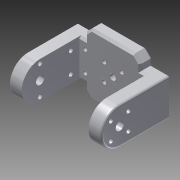
# Autodesk Inventor part: サーボ首不利
Saved by Autodesk Inventor 2015 (Build 190159000, 159)
## iProperties
Created: 2015-05-13
Part Number: サーボ首不利
Material: PVC、軟質
Document SubType Name: Modeling
Designer: kenta
Density: 1.3 g/cm^3
Appearance: PVC - 白
Mass: 15.4827 g
Surface Area: 60.3665 cm^2
Volume: 11.9097 cm^3
Author: kenta
Autodesk Inventor part; units mm, degrees
note: some values were not read from the file. Chosen so that the rebuilt part matches the saved one: direction of "穴4"; direction of "穴5"; direction of "穴6"; direction of "穴7"; direction of "穴8".
ref_plane "YZ Plane" through (0, 0, 0) normal (1, 0, 0) x (0, 1, 0)
ref_plane "XZ Plane" through (0, 0, 0) normal (0, 1, 0) x (-1, 0, 0)
ref_plane "XY Plane" through (0, 0, 0) normal (0, 0, 1) x (1, 0, 0)
sketch "スケッチ1" plane through (0, 0, 0) normal (0, 0, 1) x (1, 0, 0)
  line L0 (-22.5, 17) -> (22.5, 17)
  line L1 (22.5, 17) -> (22.5, -17)
  line L2 (22.5, -17) -> (-22.5, -17)
  line L3 (-22.5, -17) -> (-22.5, 17)
  line L4 (-22.5, 17) -> (22.5, -17) construction
  line L5 (22.5, 17) -> (-22.5, -17) construction
  point P0 (0, 0)
  dimension "d0" = 45
  dimension "d1" = 34
  constraints: 12 end point, 2 midpoint, 2 parallel, 1 horizontal, 1 perpendicular
  measures "d0" distance of L1.end L2.end
  measures "d1" distance of L0.end L1.end
extrude "押し出し1" add sketch "スケッチ1" along normal blind 18
sketch "スケッチ2" plane through (0, 0, 18) normal (0, 0, 1) x (1, 0, 0)
  line L0 (-16.25, 11) -> (16.25, 11)
  line L1 (16.25, 11) -> (16.25, -17)
  line L2 (16.25, -17) -> (-16.25, -17)
  line L3 (-16.25, -17) -> (-16.25, 11)
  line L4 (-22.5, 17) -> (-22.5, -17) projected
  line L5 (22.5, -17) -> (22.5, 17) projected
  line L6 (22.5, 17) -> (-22.5, 17) projected
  line L7 (-22.5, -17) -> (22.5, -17) projected
  point P0 (0, 0)
  dimension "d4" = 6.25
  dimension "d5" = 6.25
  dimension "d6" = 6
  dimension "d7" = 0
  constraints: 8 end point, 2 parallel, 1 horizontal, 1 perpendicular
  measures "d4" distance between parallel lines of L3 L4
  measures "d5" distance between parallel lines of L5 L1
  measures "d6" distance between parallel lines of L6 L0
  measures "d7" distance between parallel lines of L7 L2
extrude "押し出し2" cut sketch "スケッチ2" against normal blind 18 contours L0 L1 L2 L3
sketch "スケッチ4" plane through (22.5, -17, 0) normal (1, 0, 0) x (0, 0, -1)
  line L0 (0, 34) -> (-18, 34) projected
  point P0 (0, 17)
  point P1 (-9, 9)
  dimension "d17" = 25
  measures "d17" distance from line of point (-9, 9) L0
hole "穴1" at (22.5, -8, 9) direction (-1, 0, 0) diameter 4 end through all
fillet "フィレット1" radius 9 6 edges at (19.375, -17, 0) (19.375, -17, 18) (22.5, -17, 9) (-22.5, -17, 9) (-19.375, -17, 0) (-19.375, -17, 18)
fillet "フィレット2" radius 1 6 edges at (-22.5, 4.5, 0) (-22.5, 4.5, 18) (-22.5, -17, 9) (22.5, 4.5, 18) (22.5, 4.5, 0) (22.5, -17, 9)
sketch "スケッチ5" plane through (-21.5, 17, 0) normal (0, 1, 0) x (1, 0, 0)
  point P0 (21.5, 0)
  point P1 (21.5, -9)
  dimension "d65" = 0
  measures "d65" horizontal distance of point (21.5, 0) point (21.5, -9)
hole "穴2" at (0, 17, 9) direction (0, -1, 0) diameter 3 end through all
sketch "スケッチ7" plane through (22.5, -8, 1) normal (1, 0, 0) x (0, 0, -1)
  circle A0 centre (-8, 0) radius 2 projected
  line L0 (-8, 0) -> (-12.2426, -4.2426)
  line L1 (-8, 0) -> (-2, 0) construction
  point P0 (1, 8)
  dimension "d40" = 6
  dimension "d41" = 135
  constraints: 4 end point, 1 coincident, 1 equal length, 1 horizontal
  measures "d40" distance of L0.start L0.end
  measures "d41" angle of L0 L1
hole "穴4" at (22.5, -12.2426, 13.2426) direction (-1, 0, 0) diameter 2 end up to surface
pattern_circular "円形状パターン1" count 4 over 360 about axis through (-36.703, -8, 9) along (1, 0, 0) of "穴4"
sketch "スケッチ8" plane through (0, 0, 18) normal (0, 0, 1) x (1, 0, 0)
  line L0 (-16.25, 11) -> (16.25, 11) projected
  line L1 (13.5, 23) -> (-13.5, 23)
  line L2 (-13.5, 23) -> (-13.5, 11)
  line L3 (-13.5, 11) -> (13.5, 11)
  line L4 (13.5, 11) -> (13.5, 23)
  line L5 (21.5, 17) -> (-21.5, 17) projected
  line L6 (13.5, 23) -> (-13.5, 11) construction
  line L7 (-13.5, 23) -> (13.5, 11) construction
  line L8 (13.5, 17) -> (13.5, 11)
  line L9 (13.5, 11) -> (-13.5, 11)
  line L10 (-13.5, 11) -> (-13.5, 17)
  line L11 (13.5, 17) -> (13.5, 11)
  line L12 (13.5, 11) -> (-13.5, 11)
  line L13 (-13.5, 17) -> (13.5, 17)
  point P0 (0, 0)
  point P1 (0, 17)
  dimension "d52" = 27
  constraints: 24 end point, 5 midpoint, 3 collinear, 3 perpendicular, 3 point on line, 2 parallel, 1 horizontal
  measures "d52" distance of L3.end L2.end
extrude "押し出し3" add sketch "スケッチ8" along normal blind 6 contours L2 L5 L4 L0
sketch "スケッチ9" plane through (0, 0, 0) normal (0, 0, -1) x (-1, 0, 0)
  line L0 (21.5, 17) -> (-21.5, 17) projected
  line L1 (0, 17) -> (13.5, 17)
  line L2 (0, 17) -> (13.5, 17) construction
  line L3 (13.5, 17) -> (13.5, 11)
  line L4 (13.5, 11) -> (-13.5, 11)
  line L5 (-13.5, 11) -> (-13.5, 17)
  line L6 (-13.5, 17) -> (13.5, 17)
  point P0 (0, 0)
  dimension "d55" = 13.5
  dimension "d56" = 0
  dimension "d57" = 27
  dimension "d58" = 6
  dimension "d59" = 90
  constraints: 12 end point, 2 collinear, 1 horizontal, 1 midpoint, 1 perpendicular
  measures "d55" distance of L1.start L1.end
  measures "d56" distance between parallel lines of L1 L2
  measures "d57" distance of L3.end L4.end
  measures "d58" distance of L4.end L5.end
  measures "d59" angle of L4 L5
extrude "押し出し4" add sketch "スケッチ9" along normal blind 6
chamfer "面取り1" distance 3 angle 45 4 edges at (-13.5, 14, 24) (13.5, 14, 24) (13.5, 14, -6) (-13.5, 14, -6)
chamfer "面取り2" distance 1 angle 45 20 edges at (0, 17, -6) (12, 17, -4.5) (13.5, 17, -1.5) (-12, 17, -4.5) (-13.5, 17, -1.5) (-17.5, 17, 0) (-22.2071, 17, 0.2929) (-22.5, 17, 9) (-22.2071, 17, 17.7071) (-17.5, 17, 18) (17.5, 17, 0) (22.2071, 17, 0.2929) (22.5, 17, 9) (22.2071, 17, 17.7071) (17.5, 17, 18) (13.5, 17, 19.5) (12, 17, 22.5) (0, 17, 24) (-12, 17, 22.5) (-13.5, 17, 19.5)
sketch "スケッチ10" plane through (-22.5, -8, 9) normal (-1, 0, 0) x (0, 0, 1)
  point P0 (-9, 8)
  point P1 (7, 0)
  point P2 (-7, 0)
hole "穴5" at (-22.5, -8, 16) at (-22.5, -8, 2) direction (1, 0, 0) diameter 2 end up to surface
sketch "スケッチ11" plane through (-22.5, 16, 1) normal (-1, 0, 0) x (0, 0, 1)
  line L0 (-1, 0) -> (-1, -24) projected
  line L1 (17, -24) -> (17, 0) projected
  line L2 (16, 1) -> (0, 1) projected
  point P0 (-1, -16)
  point P1 (13, -9)
  point P2 (3, -9)
  dimension "d78" = 10
  dimension "d79" = 4
  dimension "d80" = 4
  dimension "d81" = 10
  constraints: 1 horizontal alignment
  measures "d78" distance of point (3, -9) point (13, -9)
  measures "d79" distance from line of point (3, -9) L0
  measures "d80" distance from line of point (13, -9) L1
  measures "d81" distance from line of point (13, -9) L2
hole "穴6" at (-22.5, 7, 14) at (-22.5, 7, 4) direction (1, 0, 0) diameter 2 end up to surface
sketch "スケッチ12" plane through (-10.0858, 17, -5) normal (0, 1, 0) x (1, 0, 0)
  line L0 (-3.4142, -5) -> (-11.4142, -5) projected
  line L1 (-11.4142, -23) -> (-3.4142, -23) projected
  line L2 (31.5858, -5) -> (23.5858, -5) projected
  point P0 (10.0858, -5)
  point P1 (-3.4142, -9)
  point P2 (-3.4142, -19)
  point P3 (23.5858, -9)
  point P4 (23.5858, -19)
  dimension "d91" = 10
  dimension "d92" = 13.5
  dimension "d93" = 10
  dimension "d94" = 13.5
  dimension "d95" = 4
  dimension "d96" = 4
  dimension "d97" = 4
  constraints: 2 vertical alignment
  measures "d91" distance of point (-3.414, -19) point (-3.414, -9)
  measures "d92" horizontal distance of point (-3.414, -9) point (10.086, -5)
  measures "d93" distance of point (23.586, -19) point (23.586, -9)
  measures "d94" horizontal distance of point (23.586, -9) point (10.086, -5)
  measures "d95" distance from line of point (-3.414, -9) L0
  measures "d96" distance from line of point (-3.414, -19) L1
  measures "d97" distance from line of point (23.586, -9) L2
hole "穴7" at (-13.5, 17, 4) at (-13.5, 17, 14) at (13.5, 17, 4) at (13.5, 17, 14) direction (0, -1, 0) diameter 2 end up to surface
sketch "スケッチ13" plane through (-10.0858, 17, -5) normal (0, 1, 0) x (1, 0, 0)
  circle A0 centre (10.0858, -14) radius 1.5 projected
  line L0 (10.0858, -14) -> (5.8431, -9.7574)
  line L1 (10.0858, -14) -> (16.0858, -14) construction
  point P0 (10.0858, -5)
  point P1 (5.8546, -9.7688)
  dimension "d105" = 6
  dimension "d106" = 135
  constraints: 4 end point, 1 equal length, 1 horizontal, 1 point on line
  measures "d105" distance of L0.start L0.end
  measures "d106" angle of L1 L0
hole "穴8" at (-4.2312, 17, 4.7688) direction (0, -1, 0) diameter 2 end up to surface
pattern_circular "円形状パターン2" count 4 over 360 about axis through (0, -42.203, 9) along (0, 1, 0) of "穴8"
chamfer "面取り3" distance 1 angle 45 14 edges at (0, 11, -6) (-12, 11, -4.5) (-13.5, 11, -1.5) (-14.875, 11, 0) (12, 11, -4.5) (13.5, 11, -1.5) (14.875, 11, 0) (0, 11, 24) (-12, 11, 22.5) (-13.5, 11, 19.5) (-14.875, 11, 18) (12, 11, 22.5) (13.5, 11, 19.5) (14.875, 11, 18)
